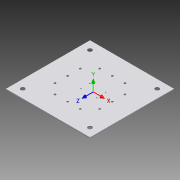
# Autodesk Inventor part: BottomBasePlate
Saved by Autodesk Inventor 2015 (Build 190159000, 159)
## iProperties
Created: 2014-05-24
Part Number: BottomBasePlate
Material: Aluminum 6061
Document SubType Name: Sheet Metal
Designer: seaha_000
Density: 2.7 g/cm^3
Sheet Metal Rule: 1/8in Aluminium
Appearance: Aluminum - Flat
Mass: 545.102 g
Surface Area: 1318.13 cm^2
Volume: 201.889 cm^3
Author: seaha_000
Autodesk Inventor part; units mm, degrees
ref_plane "YZ Plane" through (0, 0, 0) normal (1, 0, 0) x (0, 1, 0)
ref_plane "XZ Plane" through (0, 0, 0) normal (0, 1, 0) x (-1, 0, 0)
ref_plane "XY Plane" through (0, 0, 0) normal (0, 0, 1) x (1, 0, 0)
sketch "Sketch1" plane through (0, 0, 0) normal (0, 1, 0) x (-1, 0, 0)
  line L0 (-2.2451, 151.7551) -> (-2.2451, 2.2451)
  line L1 (16.8049, 21.2951) -> (-2.2451, 2.2451)
  line L2 (16.8049, 132.7051) -> (16.8049, 21.2951)
  line L3 (-2.2451, 151.7551) -> (16.8049, 132.7051)
  line L4 (0, 0) -> (149.5101, 0)
  line L5 (130.4601, 19.05) -> (149.5101, 0)
  line L6 (19.05, 19.05) -> (130.4601, 19.05)
  line L7 (0, 0) -> (19.05, 19.05)
  line L8 (151.7551, 2.2451) -> (151.7551, 151.7551)
  line L9 (132.7051, 132.7051) -> (151.7551, 151.7551)
  line L10 (132.7051, 21.2951) -> (132.7051, 132.7051)
  line L11 (151.7551, 2.2451) -> (132.7051, 21.2951)
  line L12 (149.5101, 154.0002) -> (0, 154.0002)
  line L13 (19.05, 134.9502) -> (0, 154.0002)
  line L14 (130.4601, 134.9502) -> (19.05, 134.9502)
  line L15 (149.5101, 154.0002) -> (130.4601, 134.9502)
  line L16 (9.525, 144.4752) -> (139.9851, 144.4752) construction
  line L17 (149.5101, 154.0002) -> (130.4601, 134.9502) construction
  line L18 (151.7551, 151.7551) -> (132.7051, 132.7051) construction
  line L19 (142.2301, 142.2301) -> (142.2301, 11.7701) construction
  line L20 (130.4601, 19.05) -> (149.5101, 0) construction
  line L21 (139.9851, 9.525) -> (9.525, 9.525) construction
  line L22 (0, 0) -> (19.05, 19.05) construction
  line L23 (-2.2451, 2.2451) -> (16.8049, 21.2951) construction
  line L24 (7.2799, 11.7701) -> (7.2799, 142.2301) construction
  circle A0 centre (142.2301, 77.0001) radius 3.175
  circle A1 centre (74.755, 9.525) radius 3.175
  circle A2 centre (7.2799, 77.0001) radius 3.175
  circle A3 centre (74.755, 144.4752) radius 3.175
  circle A4 centre (112.855, 144.4752) radius 3.175
  circle A5 centre (36.655, 144.4752) radius 3.175
  circle A6 centre (74.755, 144.4752) radius 3.175
  circle A7 centre (7.2799, 38.9001) radius 3.175
  circle A8 centre (7.2799, 115.1001) radius 3.175
  circle A9 centre (7.2799, 77.0001) radius 3.175
  circle A10 centre (142.2301, 115.1001) radius 3.175
  circle A11 centre (142.2301, 38.9001) radius 3.175
  circle A12 centre (142.2301, 77.0001) radius 3.175
  circle A13 centre (36.655, 9.525) radius 3.175
  circle A14 centre (112.855, 9.525) radius 3.175
  circle A15 centre (74.755, 9.525) radius 3.175
  circle A16 centre (74.755, 77.0001) radius 57.9501 construction
  line L25 (-52.245, 204.0001) -> (201.755, 204.0001)
  line L26 (201.755, 204.0001) -> (201.755, -49.9999)
  line L27 (201.755, -49.9999) -> (-52.245, -49.9999)
  line L28 (-52.245, -49.9999) -> (-52.245, 204.0001)
  line L29 (-52.245, 204.0001) -> (201.755, -49.9999) construction
  line L30 (201.755, 204.0001) -> (-52.245, -49.9999) construction
  point P0 (151.7551, 0)
  dimension "d16" = 19.05
  dimension "d17" = 19.05
  dimension "d18" = 19.05
  dimension "d19" = 19.05
  dimension "d20" = 6.35
  dimension "d21" = 6.35
  dimension "d22" = 6.35
  dimension "d23" = 6.35
  dimension "d24" = 65.23
  dimension "d25" = 9.525
  dimension "d26" = 38.1
  dimension "d27" = 38.1
  dimension "d28" = 38.1
  dimension "d29" = 38.1
  dimension "d30" = 38.1
  dimension "d31" = 38.1
  dimension "d32" = 38.1
  dimension "d33" = 38.1
  dimension "d34" = 90
  dimension "d35" = 45
  dimension "d36" = 90
  dimension "d37" = 90
  dimension "d38" = 90
  dimension "d39" = 3.175
  dimension "d40" = 19.05
  dimension "d41" = 19.05
  dimension "d42" = 134.9502
  dimension "d43" = 154.0002
  dimension "d44" = 288.9504
  dimension "d45" = 154.0002
  dimension "d46" = 6.35
  dimension "d47" = 0
  dimension "d48" = 108.8946
  dimension "d49" = 151.7551
  dimension "d50" = 154.0002
  dimension "d51" = 6.35
  dimension "d52" = 211.4392
  dimension "d53" = 108.8946
  dimension "d54" = 3.175
  dimension "d55" = 214.6142
  dimension "d56" = 1.5875
  dimension "d57" = 254
  dimension "d58" = 254
  measures "d16" diameter of L2 L24
  measures "d17" diameter of L6 L21
  measures "d18" diameter of L12 L16
  measures "d19" diameter of L8 L19
  measures "d20" diameter of A0
  measures "d21" diameter of A1
  measures "d22" diameter of A2
  measures "d23" diameter of A3
  measures "d24" distance of L16.start A3.centre
  measures "d25" distance from line of L12 A3.centre
  measures "d26" distance of A3.centre A4.centre
  measures "d27" distance of A3.centre A5.centre
  measures "d28" distance of A2.centre A7.centre
  measures "d29" distance of A2.centre A8.centre
  measures "d30" distance of A0.centre A10.centre
  measures "d31" distance of A0.centre A11.centre
  measures "d32" distance of A1.centre A13.centre
  measures "d33" distance of A1.centre A14.centre
  measures "d34" angle of L18 L11
  measures "d35" angle of L18 L8
  measures "d36" angle of L18 L20
  measures "d37" angle of L18 L13
  measures "d38" angle of L11 L17
  measures "d39" distance between parallel lines of L11 L3
  measures "d40" diameter of L8 L19
  measures "d41" distance between parallel lines of L10 L8
  measures "d42" distance between parallel lines of L2 L8
  measures "d43" distance between parallel lines of L0 L8
  measures "d44" diameter of L12 L21
  measures "d45" distance between parallel lines of L4 L12
  measures "d46" diameter of L1 L22
  measures "d47" distance from line of point (0, 0) L18
  measures "d48" distance from line of point (0, 0) L11
  measures "d49" distance from line of point (0, 0) L8
  measures "d50" distance from line of point (0, 0) L12
  measures "d51" diameter of point (0, 0) L17
  measures "d52" diameter of point (0, 0) L20
  measures "d53" distance from line of point (0, 0) L13
  measures "d54" distance from line of point (0, 0) L1
  measures "d55" diameter of point (151.755, 0) L18
  measures "d56" distance from line of point (151.755, 0) L11
  measures "d57" distance of L25.end L26.end
  measures "d58" distance of L25.start L25.end
extrude "Plate1" add sketch "Sketch1" along normal blind 3.175 contours L3 L2 L1 L0 | L7 L6 L5 L4 | L11 L10 L9 L8 | L15 L14 L13 L12 | L25 L26 L27 L28
sketch "Sketch2" plane through (0, 3.175, 0) normal (0, 1, 0) x (1, 0, 0)
  line L0 (-201.755, 49.9999) -> (52.245, 49.9999) projected
  line L1 (-201.755, -204.0001) -> (-201.755, 49.9999) projected
  line L2 (52.245, -204.0001) -> (-201.755, -204.0001) projected
  line L3 (52.245, 49.9999) -> (52.245, -204.0001) projected
  line L4 (26.845, 24.5999) -> (-176.355, 24.5999)
  line L5 (-176.355, 24.5999) -> (-176.355, -178.6001)
  line L6 (-176.355, -178.6001) -> (26.845, -178.6001)
  line L7 (26.845, -178.6001) -> (26.845, 24.5999)
  circle A0 centre (-176.355, 24.5999) radius 6.35
  circle A1 centre (26.845, 24.5999) radius 6.35
  circle A2 centre (-176.355, -178.6001) radius 6.35
  circle A3 centre (26.845, -178.6001) radius 6.35
  point P0 (0, 0)
  dimension "d60" = 203.2
  dimension "d61" = 12.7
  dimension "d62" = 12.7
  dimension "d63" = 12.7
  dimension "d64" = 12.7
  constraints: 8 end point, 4 centre point, 4 coincident, 3 other
  measures "d60" distance of L4.start L4.end
  measures "d61" diameter of A0
  measures "d62" diameter of A1
  measures "d63" diameter of A2
  measures "d64" diameter of A3
extrude "Cut1" cut sketch "Sketch2" against normal blind 3.175 contours A0 L5 L4 | L4 L5 A0 | A1 L7 L4 | L4 L7 A1 | A2 L6 L5 | L5 L6 A2 | A3 L6 L7 | L7 L6 A3
sketch "Sketch7" plane through (-64.7482, 0, 77.0128) normal (0, 1, 0) x (0, 0, 1)
  line L0 (15.2484, -23.8801) -> (15.2484, -22.1021)
  arc A0 (11.6924, -23.8801) -> (15.2484, -23.8801) centre (13.4704, -23.8801) ccw
  line L1 (11.6924, -22.1021) -> (11.6924, -23.8801)
  arc A1 (15.2484, -22.1021) -> (11.6924, -22.1021) centre (13.4704, -22.1021) ccw
  line L2 (11.6924, 23.8801) -> (11.6924, 22.1021)
  arc A2 (15.2484, 23.8801) -> (11.6924, 23.8801) centre (13.4704, 23.8801) ccw
  line L3 (15.2484, 22.1021) -> (15.2484, 23.8801)
  arc A3 (11.6924, 22.1021) -> (15.2484, 22.1021) centre (13.4704, 22.1021) ccw
  line L4 (11.6924, 15.9807) -> (11.6924, 14.2027)
  arc A4 (15.2484, 15.9807) -> (11.6924, 15.9807) centre (13.4704, 15.9807) ccw
  line L5 (15.2484, 14.2027) -> (15.2484, 15.9807)
  arc A5 (11.6924, 14.2027) -> (15.2484, 14.2027) centre (13.4704, 14.2027) ccw
  line L6 (15.2484, 3.0607) -> (15.2484, 4.8387)
  arc A6 (11.6924, 3.0607) -> (15.2484, 3.0607) centre (13.4704, 3.0607) ccw
  line L7 (11.6924, 4.8387) -> (11.6924, 3.0607)
  arc A7 (15.2484, 4.8387) -> (11.6924, 4.8387) centre (13.4704, 4.8387) ccw
  line L8 (15.2484, -4.8387) -> (15.2484, -3.0607)
  arc A8 (11.6924, -4.8387) -> (15.2484, -4.8387) centre (13.4704, -4.8387) ccw
  line L9 (11.6924, -3.0607) -> (11.6924, -4.8387)
  arc A9 (15.2484, -3.0607) -> (11.6924, -3.0607) centre (13.4704, -3.0607) ccw
  line L10 (15.2484, -15.9807) -> (15.2484, -14.2027)
  arc A10 (11.6924, -15.9807) -> (15.2484, -15.9807) centre (13.4704, -15.9807) ccw
  line L11 (11.6924, -14.2027) -> (11.6924, -15.9807)
  arc A11 (15.2484, -14.2027) -> (11.6924, -14.2027) centre (13.4704, -14.2027) ccw
  line L12 (-15.2484, 23.8801) -> (-15.2484, 22.1021)
  arc A12 (-11.6924, 23.8801) -> (-15.2484, 23.8801) centre (-13.4704, 23.8801) ccw
  line L13 (-11.6924, 22.1021) -> (-11.6924, 23.8801)
  arc A13 (-15.2484, 22.1021) -> (-11.6924, 22.1021) centre (-13.4704, 22.1021) ccw
  line L14 (-15.2484, 15.9807) -> (-15.2484, 14.2027)
  arc A14 (-11.6924, 15.9807) -> (-15.2484, 15.9807) centre (-13.4704, 15.9807) ccw
  line L15 (-11.6924, 14.2027) -> (-11.6924, 15.9807)
  arc A15 (-15.2484, 14.2027) -> (-11.6924, 14.2027) centre (-13.4704, 14.2027) ccw
  line L16 (-11.6924, 3.0607) -> (-11.6924, 4.8387)
  arc A16 (-15.2484, 3.0607) -> (-11.6924, 3.0607) centre (-13.4704, 3.0607) ccw
  line L17 (-15.2484, 4.8387) -> (-15.2484, 3.0607)
  arc A17 (-11.6924, 4.8387) -> (-15.2484, 4.8387) centre (-13.4704, 4.8387) ccw
  line L18 (-11.6924, -4.8387) -> (-11.6924, -3.0607)
  arc A18 (-15.2484, -4.8387) -> (-11.6924, -4.8387) centre (-13.4704, -4.8387) ccw
  line L19 (-15.2484, -3.0607) -> (-15.2484, -4.8387)
  arc A19 (-11.6924, -3.0607) -> (-15.2484, -3.0607) centre (-13.4704, -3.0607) ccw
  line L20 (-11.6924, -15.9807) -> (-11.6924, -14.2027)
  arc A20 (-15.2484, -15.9807) -> (-11.6924, -15.9807) centre (-13.4704, -15.9807) ccw
  line L21 (-15.2484, -14.2027) -> (-15.2484, -15.9807)
  arc A21 (-11.6924, -14.2027) -> (-15.2484, -14.2027) centre (-13.4704, -14.2027) ccw
  line L22 (-11.6924, -23.8801) -> (-11.6924, -22.1021)
  arc A22 (-15.2484, -23.8801) -> (-11.6924, -23.8801) centre (-13.4704, -23.8801) ccw
  line L23 (-15.2484, -22.1021) -> (-15.2484, -23.8801)
  arc A23 (-11.6924, -22.1021) -> (-15.2484, -22.1021) centre (-13.4704, -22.1021) ccw
  arc A24 (6.3525, -24) -> (3.6475, -24) centre (5, -24) ccw
  arc A25 (3.6475, -24) -> (6.3525, -24) centre (5, -24) ccw
  arc A26 (6.3525, 24) -> (3.6475, 24) centre (5, 24) ccw
  arc A27 (3.6475, 24) -> (6.3525, 24) centre (5, 24) ccw
  line L24 (-10.16, 20.828) -> (-10.16, -20.828)
  arc A28 (-6.096, 20.828) -> (-10.16, 20.828) centre (-8.128, 20.828) ccw
  line L25 (-2.3813, 20.828) -> (-6.096, 20.828)
  line L26 (-2.3813, 25.908) -> (-2.3813, 20.828)
  arc A29 (2.3812, 25.908) -> (-2.3813, 25.908) centre (0, 25.908) ccw
  line L27 (2.3812, 20.828) -> (2.3812, 25.908)
  line L28 (6.096, 20.828) -> (2.3812, 20.828)
  arc A30 (10.16, 20.828) -> (6.096, 20.828) centre (8.128, 20.828) ccw
  line L29 (10.16, -20.828) -> (10.16, 20.828)
  arc A31 (6.096, -20.828) -> (10.16, -20.828) centre (8.128, -20.828) ccw
  line L30 (2.3813, -20.828) -> (6.096, -20.828)
  line L31 (2.3813, -25.908) -> (2.3813, -20.828)
  arc A32 (-2.3812, -25.908) -> (2.3813, -25.908) centre (0, -25.908) ccw
  line L32 (-2.3813, -20.828) -> (-2.3812, -25.908)
  line L33 (-6.096, -20.828) -> (-2.3813, -20.828)
  arc A33 (-10.16, -20.828) -> (-6.096, -20.828) centre (-8.128, -20.828) ccw
  arc A34 (-4.572, -28.448) -> (4.572, -28.448) centre (0, -24.8232) ccw
  line L34 (4.572, -28.448) -> (13.462, -28.448)
  arc A35 (13.462, -28.448) -> (16.637, -25.273) centre (13.462, -25.273) ccw
  line L35 (16.637, -25.273) -> (16.637, 25.273)
  arc A36 (16.637, 25.273) -> (13.462, 28.448) centre (13.462, 25.273) ccw
  line L36 (13.462, 28.448) -> (4.572, 28.448)
  arc A37 (4.572, 28.448) -> (-4.572, 28.448) centre (0, 24.8232) ccw
  line L37 (-4.572, 28.448) -> (-13.462, 28.448)
  arc A38 (-13.462, 28.448) -> (-16.637, 25.273) centre (-13.462, 25.273) ccw
  line L38 (-16.637, 25.273) -> (-16.637, -25.273)
  arc A39 (-16.637, -25.273) -> (-13.462, -28.448) centre (-13.462, -25.273) ccw
  line L39 (-13.462, -28.448) -> (-4.572, -28.448)
  arc A40 (-3.6475, 24) -> (-6.3525, 24) centre (-5, 24) ccw
  arc A41 (-6.3525, 24) -> (-3.6475, 24) centre (-5, 24) ccw
  arc A42 (-3.6475, -24) -> (-6.3525, -24) centre (-5, -24) ccw
  arc A43 (-6.3525, -24) -> (-3.6475, -24) centre (-5, -24) ccw
  line L40 (15.2484, -23.8801) -> (15.2484, -22.1021)
  arc A44 (11.6924, -23.8801) -> (15.2484, -23.8801) centre (13.4704, -23.8801) ccw
  line L41 (11.6924, -22.1021) -> (11.6924, -23.8801)
  arc A45 (15.2484, -22.1021) -> (11.6924, -22.1021) centre (13.4704, -22.1021) ccw
  line L42 (11.6924, 23.8801) -> (11.6924, 22.1021)
  arc A46 (15.2484, 23.8801) -> (11.6924, 23.8801) centre (13.4704, 23.8801) ccw
  line L43 (15.2484, 22.1021) -> (15.2484, 23.8801)
  arc A47 (11.6924, 22.1021) -> (15.2484, 22.1021) centre (13.4704, 22.1021) ccw
  line L44 (11.6924, 15.9807) -> (11.6924, 14.2027)
  arc A48 (15.2484, 15.9807) -> (11.6924, 15.9807) centre (13.4704, 15.9807) ccw
  line L45 (15.2484, 14.2027) -> (15.2484, 15.9807)
  arc A49 (11.6924, 14.2027) -> (15.2484, 14.2027) centre (13.4704, 14.2027) ccw
  line L46 (15.2484, 3.0607) -> (15.2484, 4.8387)
  arc A50 (11.6924, 3.0607) -> (15.2484, 3.0607) centre (13.4704, 3.0607) ccw
  line L47 (11.6924, 4.8387) -> (11.6924, 3.0607)
  arc A51 (15.2484, 4.8387) -> (11.6924, 4.8387) centre (13.4704, 4.8387) ccw
  line L48 (15.2484, -4.8387) -> (15.2484, -3.0607)
  arc A52 (11.6924, -4.8387) -> (15.2484, -4.8387) centre (13.4704, -4.8387) ccw
  line L49 (11.6924, -3.0607) -> (11.6924, -4.8387)
  arc A53 (15.2484, -3.0607) -> (11.6924, -3.0607) centre (13.4704, -3.0607) ccw
  line L50 (15.2484, -15.9807) -> (15.2484, -14.2027)
  arc A54 (11.6924, -15.9807) -> (15.2484, -15.9807) centre (13.4704, -15.9807) ccw
  line L51 (11.6924, -14.2027) -> (11.6924, -15.9807)
  arc A55 (15.2484, -14.2027) -> (11.6924, -14.2027) centre (13.4704, -14.2027) ccw
  line L52 (-15.2484, 23.8801) -> (-15.2484, 22.1021)
  arc A56 (-11.6924, 23.8801) -> (-15.2484, 23.8801) centre (-13.4704, 23.8801) ccw
  line L53 (-11.6924, 22.1021) -> (-11.6924, 23.8801)
  arc A57 (-15.2484, 22.1021) -> (-11.6924, 22.1021) centre (-13.4704, 22.1021) ccw
  line L54 (-15.2484, 15.9807) -> (-15.2484, 14.2027)
  arc A58 (-11.6924, 15.9807) -> (-15.2484, 15.9807) centre (-13.4704, 15.9807) ccw
  line L55 (-11.6924, 14.2027) -> (-11.6924, 15.9807)
  arc A59 (-15.2484, 14.2027) -> (-11.6924, 14.2027) centre (-13.4704, 14.2027) ccw
  line L56 (-11.6924, 3.0607) -> (-11.6924, 4.8387)
  arc A60 (-15.2484, 3.0607) -> (-11.6924, 3.0607) centre (-13.4704, 3.0607) ccw
  line L57 (-15.2484, 4.8387) -> (-15.2484, 3.0607)
  arc A61 (-11.6924, 4.8387) -> (-15.2484, 4.8387) centre (-13.4704, 4.8387) ccw
  line L58 (-11.6924, -4.8387) -> (-11.6924, -3.0607)
  arc A62 (-15.2484, -4.8387) -> (-11.6924, -4.8387) centre (-13.4704, -4.8387) ccw
  line L59 (-15.2484, -3.0607) -> (-15.2484, -4.8387)
  arc A63 (-11.6924, -3.0607) -> (-15.2484, -3.0607) centre (-13.4704, -3.0607) ccw
  line L60 (-11.6924, -15.9807) -> (-11.6924, -14.2027)
  arc A64 (-15.2484, -15.9807) -> (-11.6924, -15.9807) centre (-13.4704, -15.9807) ccw
  line L61 (-15.2484, -14.2027) -> (-15.2484, -15.9807)
  arc A65 (-11.6924, -14.2027) -> (-15.2484, -14.2027) centre (-13.4704, -14.2027) ccw
  line L62 (-11.6924, -23.8801) -> (-11.6924, -22.1021)
  arc A66 (-15.2484, -23.8801) -> (-11.6924, -23.8801) centre (-13.4704, -23.8801) ccw
  line L63 (-15.2484, -22.1021) -> (-15.2484, -23.8801)
  arc A67 (-11.6924, -22.1021) -> (-15.2484, -22.1021) centre (-13.4704, -22.1021) ccw
  arc A68 (6.3525, -24) -> (3.6475, -24) centre (5, -24) ccw
  arc A69 (3.6475, -24) -> (6.3525, -24) centre (5, -24) ccw
  arc A70 (6.3525, 24) -> (3.6475, 24) centre (5, 24) ccw
  arc A71 (3.6475, 24) -> (6.3525, 24) centre (5, 24) ccw
  line L64 (-10.16, 20.828) -> (-10.16, -20.828)
  arc A72 (-6.096, 20.828) -> (-10.16, 20.828) centre (-8.128, 20.828) ccw
  line L65 (-2.3813, 20.828) -> (-6.096, 20.828)
  line L66 (-2.3813, 25.908) -> (-2.3813, 20.828)
  arc A73 (2.3812, 25.908) -> (-2.3813, 25.908) centre (0, 25.908) ccw
  line L67 (2.3812, 20.828) -> (2.3812, 25.908)
  line L68 (6.096, 20.828) -> (2.3812, 20.828)
  arc A74 (10.16, 20.828) -> (6.096, 20.828) centre (8.128, 20.828) ccw
  line L69 (10.16, -20.828) -> (10.16, 20.828)
  arc A75 (6.096, -20.828) -> (10.16, -20.828) centre (8.128, -20.828) ccw
  line L70 (2.3813, -20.828) -> (6.096, -20.828)
  line L71 (2.3813, -25.908) -> (2.3813, -20.828)
  arc A76 (-2.3812, -25.908) -> (2.3813, -25.908) centre (0, -25.908) ccw
  line L72 (-2.3813, -20.828) -> (-2.3812, -25.908)
  line L73 (-6.096, -20.828) -> (-2.3813, -20.828)
  arc A77 (-10.16, -20.828) -> (-6.096, -20.828) centre (-8.128, -20.828) ccw
  arc A78 (-4.572, -28.448) -> (4.572, -28.448) centre (0, -24.8232) ccw
  line L74 (4.572, -28.448) -> (13.462, -28.448)
  arc A79 (13.462, -28.448) -> (16.637, -25.273) centre (13.462, -25.273) ccw
  line L75 (16.637, -25.273) -> (16.637, 25.273)
  arc A80 (16.637, 25.273) -> (13.462, 28.448) centre (13.462, 25.273) ccw
  line L76 (13.462, 28.448) -> (4.572, 28.448)
  arc A81 (4.572, 28.448) -> (-4.572, 28.448) centre (0, 24.8232) ccw
  line L77 (-4.572, 28.448) -> (-13.462, 28.448)
  arc A82 (-13.462, 28.448) -> (-16.637, 25.273) centre (-13.462, 25.273) ccw
  line L78 (-16.637, 25.273) -> (-16.637, -25.273)
  arc A83 (-16.637, -25.273) -> (-13.462, -28.448) centre (-13.462, -25.273) ccw
  line L79 (-13.462, -28.448) -> (-4.572, -28.448)
  arc A84 (-3.6475, 24) -> (-6.3525, 24) centre (-5, 24) ccw
  arc A85 (-6.3525, 24) -> (-3.6475, 24) centre (-5, 24) ccw
  arc A86 (-3.6475, -24) -> (-6.3525, -24) centre (-5, -24) ccw
  arc A87 (-6.3525, -24) -> (-3.6475, -24) centre (-5, -24) ccw
  circle A88 centre (13.4704, -23.8801) radius 1.778
  circle A89 centre (13.4704, 23.8801) radius 1.778
  circle A90 centre (13.4704, -4.8387) radius 1.778
  circle A91 centre (13.4704, 4.8387) radius 1.778
  circle A92 centre (-13.4704, -23.8801) radius 1.778
  circle A93 centre (-13.4704, 23.8801) radius 1.778
  circle A94 centre (-13.4704, -4.8387) radius 1.778
  circle A95 centre (-13.4704, 4.8387) radius 1.778
  point P0 (0, 0)
  point P1 (0, 0)
  constraints: 176 point on circle, 160 end point, 96 centre point, 8 coincident
hole "Hole1" [suppressed]
sketch "Sketch8" plane through (0, 3.175, 0) normal (0, 1, 0) x (1, 0, 0)
  circle A0 centre (-88.6376, -63.5246) radius 1.778
  circle A1 centre (-88.6376, -90.4654) radius 1.778
  circle A2 centre (-40.8775, -63.5246) radius 1.778
  circle A3 centre (-40.8775, -90.4654) radius 1.778
  point P0 (0, 0)
  point P1 (-88.6376, -63.5246)
  point P2 (-88.6376, -90.4654)
  point P3 (-40.8775, -63.5246)
  point P4 (-40.8775, -90.4654)
  constraints: 4 centre point, 12 other
hole "Hole2" at (-88.6376, 3.175, 63.5246) at (-88.6376, 3.175, 90.4654) at (-40.8775, 3.175, 63.5246) at (-40.8775, 3.175, 90.4654) direction (0, -1, 0) diameter 3.6576 end through all clearance for "Flat Head Machine Screw (82)" size "#6" standard "Ansi Unified Screw Threads"
sketch "Sketch9" plane through (0, 3.175, 0) normal (0, 1, 0) x (1, 0, 0)
  circle A0 centre (-88.6376, -63.5246) radius 1.8288 projected
  circle A1 centre (-40.8775, -63.5246) radius 1.8288 projected
  circle A2 centre (-40.8775, -90.4654) radius 1.8288 projected
  circle A3 centre (-88.6376, -90.4654) radius 1.8288 projected
  line L0 (-201.755, 49.9999) -> (52.245, 49.9999) projected
  line L1 (52.245, 49.9999) -> (52.245, -204.0001) projected
  line L2 (-201.755, -204.0001) -> (-201.755, 49.9999) projected
  line L3 (52.245, -204.0001) -> (-201.755, -204.0001) projected
  point P0 (0, 0)
  dimension "d90" = 93.1224
  dimension "d91" = 113.5245
  measures "d90" distance from line of L1 A1.centre
  measures "d91" distance from line of L0 A1.centre
equation "\"d16\" = d18"
equation "\"d17\" = d16"
equation "\"d19\" = d18"
equation "\"d20\" = d23"
equation "\"d21\" = d23"
equation "\"d22\" = d23"
equation "\"d62\" = d61"
equation "\"d63\" = d61"
equation "\"d64\" = d61"
equation "\"d65\" = Thickness"
equation "\"d81\" = Thickness"
equation "\"d88\" = Thickness"
equation "\"BendRadius\" = Thickness"
equation "\"BendReliefWidth\" = Thickness"
equation "\"BendReliefDepth\" = 0.5 * Thickness"
equation "\"CornerReliefSize\" = 4 * Thickness"
equation "\"MinimumRemnant\" = 2 * Thickness"
equation "\"TransitionRadius\" = BendRadius"
equation "\"JacobiRadiusSize\" = BendRadius"
equation "\"GapSize\" = Thickness"
equation "\"d59\" = BendRadius"
equation "\"Thickness\" = 3.175"
body "Solid1"
